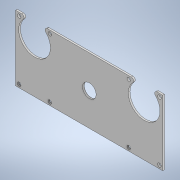
# Autodesk Inventor part: Part1
Saved by Autodesk Inventor 2020.5 (Build 245400000, 400)
## iProperties
Created: 2022-11-15
Part Number: Part1
Material: 一般
Document SubType Name: Modeling
Designer: Administrator
Density: 1 g/cm^3
Appearance: 既定
Author: Administrator
Autodesk Inventor part; units mm, degrees
ref_plane "YZ Plane" through (0, 0, 0) normal (1, 0, 0) x (0, 1, 0)
ref_plane "XZ Plane" through (0, 0, 0) normal (0, 1, 0) x (-1, 0, 0)
ref_plane "XY Plane" through (0, 0, 0) normal (0, 0, 1) x (1, 0, 0)
sketch "スケッチ1" plane through (0, 0, 0) normal (0, 0, 1) x (1, 0, 0)
  line L0 (16.5289, 13.35) -> (-12.6397, 13.35) projected
  line L1 (-12.6397, 13.35) -> (-14.4054, 11.5843) projected
  line L2 (-14.4054, 11.5843) -> (-14.4054, -42.5843) projected
  line L3 (-14.4054, -42.5843) -> (-12.6397, -44.35) projected
  line L4 (-12.6397, -44.35) -> (16.5289, -44.35) projected
  line L5 (16.5289, -44.35) -> (18.2946, -42.5843) projected
  line L6 (18.2946, -42.5843) -> (18.2946, 11.5843) projected
  line L7 (18.2946, 11.5843) -> (16.5289, 13.35) projected
  circle A0 centre (-11.5554, 10.5) radius 2.4 projected
  circle A1 centre (15.4446, -41.5) radius 2.4 projected
  circle A2 centre (-11.5554, -41.5) radius 2.4 projected
  circle A3 centre (15.4446, -10.5) radius 1.35 projected
  circle A4 centre (-11.5554, -10.5) radius 1.35 projected
  circle A5 centre (15.4446, 10.5) radius 2.4 projected
  circle A6 centre (1.9446, 0) radius 13 projected
  line L8 (86.9266, -23.7) -> (82.2766, -23.7) projected
  line L9 (82.2766, -23.7) -> (82.2766, -42.5843) projected
  line L10 (82.2766, -42.5843) -> (84.0423, -44.35) projected
  line L11 (84.0423, -44.35) -> (113.2109, -44.35) projected
  line L12 (113.2109, -44.35) -> (114.9766, -42.5843) projected
  line L13 (114.9766, -42.5843) -> (114.9766, -23.7) projected
  line L14 (114.9766, -23.7) -> (110.3266, -23.7) projected
  arc A7 (109.8266, -23.2) -> (110.3266, -23.7) centre (110.3266, -23.2) ccw projected
  line L15 (109.8266, -23.2) -> (109.8266, -21.9243) projected
  arc A8 (109.8266, -21.9243) -> (109.7973, -21.8536) centre (109.7266, -21.9243) ccw projected
  line L16 (109.7973, -21.8536) -> (106.673, -18.7293) projected
  arc A9 (106.673, -18.7293) -> (106.6023, -18.7) centre (106.6023, -18.8) ccw projected
  line L17 (106.6023, -18.7) -> (90.6508, -18.7) projected
  arc A10 (90.6508, -18.7) -> (90.5801, -18.7293) centre (90.6508, -18.8) ccw projected
  line L18 (90.5801, -18.7293) -> (87.4559, -21.8536) projected
  arc A11 (87.4559, -21.8536) -> (87.4266, -21.9243) centre (87.5266, -21.9243) ccw projected
  line L19 (87.4266, -21.9243) -> (87.4266, -23.2) projected
  arc A12 (86.9266, -23.7) -> (87.4266, -23.2) centre (86.9266, -23.2) ccw projected
  circle A13 centre (112.1266, -41.5) radius 2.4 projected
  circle A14 centre (85.1266, -41.5) radius 2.4 projected
  line L20 (82.2766, -10.3) -> (90.695, -10.3) projected
  arc A15 (94.6266, 12.3693) -> (90.695, -10.3) centre (98.6266, 0) ccw projected
  line L21 (94.6266, 13.35) -> (94.6266, 12.3693) projected
  line L22 (94.6266, 13.35) -> (84.0423, 13.35) projected
  line L23 (84.0423, 13.35) -> (82.2766, 11.5843) projected
  line L24 (82.2766, 11.5843) -> (82.2766, -10.3) projected
  circle A16 centre (85.1266, 10.5) radius 2.4 projected
  line L25 (106.5581, -10.3) -> (114.9766, -10.3) projected
  line L26 (114.9766, -10.3) -> (114.9766, 11.5843) projected
  line L27 (114.9766, 11.5843) -> (113.2109, 13.35) projected
  line L28 (113.2109, 13.35) -> (102.6266, 13.35) projected
  line L29 (102.6266, 13.35) -> (102.6266, 12.3693) projected
  arc A17 (106.5581, -10.3) -> (102.6266, 12.3693) centre (98.6266, 0) ccw projected
  circle A18 centre (112.1266, 10.5) radius 2.4 projected
  circle A19 centre (85.1266, -41.5) radius 1.3 projected
  circle A20 centre (112.1266, -41.5) radius 1.3 projected
  circle A21 centre (112.1266, 10.5) radius 1.3 projected
  circle A22 centre (85.1266, 10.5) radius 1.3 projected
  circle A23 centre (15.4446, 10.5) radius 1.3 projected
  circle A24 centre (-11.5554, 10.5) radius 1.3 projected
  circle A25 centre (-11.5554, -41.5) radius 1.3 projected
  circle A26 centre (15.4446, -41.5) radius 1.3 projected
  circle A27 centre (50.2856, -15.5391) radius 5 projected
  line L30 (-14.7585, 13.3676) -> (114.9766, 13.3676)
  line L31 (114.9766, 13.3676) -> (114.9766, -44.35)
  line L32 (114.9766, -44.35) -> (-14.7585, -44.35)
  line L33 (-14.7585, -44.35) -> (-14.7585, 13.3676)
  circle A28 centre (50.2856, -15.5391) radius 6
  circle A29 centre (85.1266, -41.5) radius 1.6
  circle A30 centre (112.1266, -41.5) radius 1.6
  circle A31 centre (112.1266, 10.5) radius 1.6
  circle A32 centre (85.1266, 10.5) radius 1.6
  circle A33 centre (-11.5554, 10.5) radius 1.6
  circle A34 centre (15.4446, 10.5) radius 1.6
  circle A35 centre (-11.5554, -41.5) radius 1.6
  circle A36 centre (15.4446, -41.5) radius 1.6
  circle A37 centre (1.9446, 0) radius 14
  circle A38 centre (98.6266, 0) radius 14
  line L34 (-14.7353, -44.35) -> (-14.4054, 13.3676)
  point P0 (0, 0)
  point P1 (13.955, 9.6197)
  point P2 (94.4663, 13.3676)
  point P3 (94.6266, 13.35)
  point P4 (84.0423, 13.35)
  point P5 (14.5843, 13.35)
  point P6 (6.1609, 13.35)
  point P7 (-2.2718, 13.35)
  point P8 (-14.5843, 13.35)
  point P9 (-16.35, 11.5843)
  point P10 (-16.35, -42.5843)
  point P11 (-12.6397, -44.35)
  point P12 (16.5289, -44.35)
  point P13 (84.0423, -44.35)
  point P14 (113.2109, -44.35)
  point P15 (114.9766, -42.5843)
  point P16 (114.9766, -23.7)
  point P17 (113.2109, 13.35)
  point P18 (102.6266, 13.35)
  point P19 (102.7868, 13.3676)
  point P20 (84.0423, -44.35)
  point P21 (113.2109, -44.35)
  point P22 (6.1048, 13.3676)
  point P23 (-2.2157, 13.3676)
  point P24 (114.9766, -42.5843)
  point P25 (114.9766, -23.7)
  point P26 (114.9766, 11.5843)
  point P27 (114.9766, -10.3)
  point P28 (106.5581, -10.3)
  dimension "d0" = 12
  dimension "d1" = 3.2
  dimension "d2" = 3.2
  dimension "d3" = 3.2
  dimension "d4" = 3.2
  dimension "d5" = 3.2
  dimension "d6" = 3.2
  dimension "d7" = 3.2
  dimension "d8" = 3.2
  dimension "d9" = 28
  dimension "d10" = 28
  constraints: 11 centre point, 10 coincident, 10 end point, 4 point on line, 2 parallel, 1 horizontal, 1 perpendicular, 1 other
  measures "d0" diameter of A28
  measures "d1" diameter of A29
  measures "d2" diameter of A30
  measures "d3" diameter of A31
  measures "d4" diameter of A32
  measures "d5" diameter of A33
  measures "d6" diameter of A34
  measures "d7" diameter of A35
  measures "d8" diameter of A36
  measures "d9" diameter of A37
  measures "d10" diameter of A38
extrude "押し出し1" add sketch "スケッチ1" along normal blind 1.5 contours L7 L6 L5 L4 L3 L2 L1 L0 A37 | L0 A37 L30 A38 L22 L23 L24 L20 L25 L31 L14 A7 L15 A8 L16 A9 L17 A10 L18 A11 L19 A12 L8 L9 L10 L32 L5 L6 L7 | L0 L1 L2 L3 L32 L34 L30 A37 | L34 L32 L33 L30 | L30 L31 L27 L28 A38 | A38 L20 L24 L23 L22 | L10 L9 L8 A12 L19 A11 L18 A10 L17 A9 L16 A8 L15 A7 L14 L13 L12 L11 | L28 L27 L26 L25 A38 | L12 L31 L32 | A0 | A1 | A2 | A3 | A4 | A5 | A13 | A14 | A16 | A18
fillet "フィレット1" radius 2 4 edges at (102.7868, 13.3676, 0.75) (94.4663, 13.3676, 0.75) (6.1048, 13.3676, 0.75) (-2.2157, 13.3676, 0.75)
